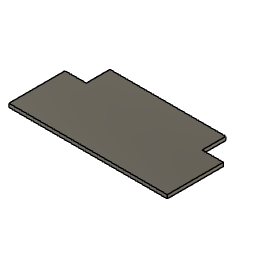
top plate v2 (Autodesk Fusion 360 design; units mm, degrees)
Autodesk Fusion 360 part; units mm, degrees
sketch "Sketch1" plane through (0, 0, 0) normal (0, 0, 1) x (1, 0, 0)
  line L0 (-56.7436, 0) -> (56.7436, 0)
  line L1 (-56.7436, 0) -> (-56.7436, 40.2082)
  line L2 (0, 5.08) -> (0, -5.08)
  line L3 (56.7436, 0) -> (56.7436, 40.2082)
  line L4 (-56.7436, 40.2082) -> (-41.529, 40.2082)
  line L5 (-41.529, 40.2082) -> (-41.529, 57.1754)
  line L6 (41.529, 40.2082) -> (41.529, 57.1754)
  line L7 (56.7436, 40.2082) -> (41.529, 40.2082)
  line L8 (-41.529, 57.1754) -> (41.529, 57.1754)
  dimension "d1" = 113.4872
  dimension "d3" = 40.2082
  dimension "d4" = 15.2146
  dimension "d5" = 16.9672
  constraint horizontal L0
  constraint perpendicular L0 L1
  constraint vertical L2
  constraint midpoint origin L2
  constraint symmetric L0.start L2 L0.end
  constraint symmetric L1.end L2 L3.end
  constraint midpoint origin L0
  constraint perpendicular L1 L4
  constraint perpendicular L4 L5
  constraint symmetric L2 L4.end L6.start
  constraint symmetric L2 L5.end L6.end
  measures "d1" distance of L0.start L0.end
  measures "d3" distance of L0.start L1.end
  measures "d4" distance of L1.end L4.end
  measures "d5" distance of L4.end L5.end
extrude "Extrude1" add sketch "Sketch1" along normal blind 2.54
